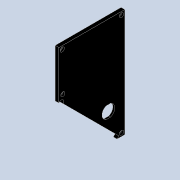
# Autodesk Inventor part: Operator Junction Box Side Panel
Saved by Autodesk Inventor 2022 (Build 260153000, 153)
## iProperties
Created: 2022-01-14
Part Number: Operator Junction Box Side Panel
Material: Generic
Document SubType Name: Modeling
Designer: Coy
Density: 1 g/cm^3
Appearance: Anodized - Black
Author: Coy
Autodesk Inventor part; units mm, degrees
ref_plane "YZ Plane" through (0, 0, 0) normal (1, 0, 0) x (0, 1, 0)
ref_plane "XZ Plane" through (0, 0, 0) normal (0, 1, 0) x (-1, 0, 0)
ref_plane "XY Plane" through (0, 0, 0) normal (0, 0, 1) x (1, 0, 0)
sketch "Sketch1" plane through (0, 0, 0) normal (1, 0, 0) x (0, 1, 0)
  circle A0 centre (7.0357, 7.0379) radius 4.5 construction
  circle A1 centre (222.967, 132.9623) radius 4.5 construction
  arc A2 (216.9926, 130.402) -> (220.4062, 126.988) centre (222.967, 132.9623) ccw construction
  arc A3 (226.4665, 117.7965) -> (220.4062, 126.988) centre (216.4665, 117.7968) ccw construction
  line L0 (226.4665, 117.7965) -> (226.4629, 22.2035) construction
  arc A4 (220.402, 13.0124) -> (226.4629, 22.2035) centre (216.4629, 22.2039) ccw construction
  arc A5 (220.402, 13.0124) -> (216.9879, 9.5985) centre (222.9623, 7.0379) ccw construction
  arc A6 (207.7966, 3.5379) -> (216.9879, 9.5985) centre (207.7966, 13.5379) ccw construction
  line L1 (207.7966, 3.5379) -> (22.2015, 3.5379) construction
  arc A7 (13.0101, 9.5985) -> (22.2015, 3.5379) centre (22.2015, 13.5379) ccw construction
  arc A8 (13.0101, 9.5985) -> (10.3808, 12.6111) centre (7.0357, 7.0379) ccw construction
  line L2 (10.3808, 12.6111) -> (3.8893, 12.6111) construction
  line L3 (3.8893, 12.6111) -> (0, 16.5)
  line L4 (0, 16.5) -> (0, 0)
  line L5 (0, 0) -> (230, 0)
  line L6 (230, 0) -> (230.0052, 140)
  line L7 (230.0052, 140) -> (127.855, 140.0038)
  arc A9 (122.0443, 130.7772) -> (127.855, 140.0038) centre (125.5635, 135.0039) ccw
  line L8 (122.0443, 130.7772) -> (119.5403, 128.2731)
  arc A10 (119.5403, 128.2731) -> (128.6878, 126.5292) centre (125.5635, 135.0039) ccw
  arc A11 (136.9343, 125.9261) -> (128.6878, 126.5292) centre (132.1469, 117.1465) ccw construction
  arc A12 (136.9343, 125.9261) -> (146.2191, 129.5969) centre (140.0462, 131.6328) ccw construction
  arc A13 (155.7163, 136.4648) -> (146.2191, 129.5969) centre (155.716, 126.4648) ccw construction
  line L9 (155.7163, 136.4648) -> (207.8014, 136.4629) construction
  arc A14 (216.9926, 130.402) -> (207.8014, 136.4629) centre (207.801, 126.4629) ccw construction
  circle A15 centre (222.9623, 7.0379) radius 4.5 construction
  circle A16 centre (140.0462, 131.6328) radius 4.5 construction
  arc A17 (184.962, 3.5379) -> (165.0484, 3.5379) centre (175.0052, 35) ccw construction
  line L10 (184.962, 3.5379) -> (226.4622, 3.5379) construction
  line L11 (226.4622, 3.5379) -> (226.4634, 35.0003) construction
  arc A18 (223.4634, 32.0004) -> (226.4634, 35.0003) centre (223.4634, 35.0004) ccw construction
  line L12 (223.4634, 32.0004) -> (213.4634, 32.0004) construction
  arc A19 (213.4634, 38.0004) -> (213.4634, 32.0004) centre (213.4634, 35.0004) ccw construction
  line L13 (213.4634, 38.0004) -> (223.4634, 38.0004) construction
  arc A20 (226.4634, 35.0003) -> (223.4634, 38.0004) centre (223.4634, 35.0004) ccw construction
  line L14 (226.4634, 35.0003) -> (226.4647, 70.0003) construction
  arc A21 (223.4647, 67.0004) -> (226.4647, 70.0003) centre (223.4647, 70.0004) ccw construction
  line L15 (223.4647, 67.0004) -> (213.4647, 67.0004) construction
  arc A22 (213.4647, 73.0004) -> (213.4647, 67.0004) centre (213.4647, 70.0004) ccw construction
  line L16 (213.4647, 73.0004) -> (223.4647, 73.0004) construction
  arc A23 (226.4647, 70.0003) -> (223.4647, 73.0004) centre (223.4647, 70.0004) ccw construction
  line L17 (226.4647, 70.0003) -> (226.466, 105.0003) construction
  arc A24 (223.466, 102.0004) -> (226.466, 105.0003) centre (223.466, 105.0004) ccw construction
  line L18 (223.466, 102.0004) -> (213.466, 102.0004) construction
  arc A25 (213.466, 108.0004) -> (213.466, 102.0004) centre (213.466, 105.0004) ccw construction
  line L19 (213.466, 108.0004) -> (223.466, 108.0004) construction
  arc A26 (226.466, 105.0003) -> (223.466, 108.0004) centre (223.466, 105.0004) ccw construction
  line L20 (226.466, 105.0003) -> (226.4672, 136.4622) construction
  line L21 (226.4672, 136.4622) -> (145.4199, 136.4652) construction
  arc A27 (145.4199, 136.4652) -> (133.0261, 129.9155) centre (145.4194, 121.4652) ccw construction
  arc A28 (119.5403, 128.2731) -> (133.0261, 129.9155) centre (125.5635, 135.0039) ccw construction
  line L22 (119.5403, 128.2731) -> (3.8893, 12.6111)
  line L23 (3.8893, 12.6111) -> (3.5357, 12.9646)
  line L24 (3.5357, 12.9646) -> (3.5357, 3.5379) construction
  line L25 (3.5357, 3.5379) -> (165.0484, 3.5379) construction
  circle A29 centre (7.0357, 7.0379) radius 2.75
  circle A30 centre (222.9623, 7.0379) radius 2.75
  circle A31 centre (222.967, 132.9623) radius 2.75
  circle A32 centre (140.0462, 131.6328) radius 2.75
  dimension "d0" = 5.5
  dimension "d1" = 5.5
  dimension "d2" = 5.5
  dimension "d3" = 5.5
  constraints: 52 end point, 50 point on circle, 33 centre point, 4 coincident
  measures "d0" diameter of A29
  measures "d1" diameter of A30
  measures "d2" diameter of A31
  measures "d3" diameter of A32
extrude "Extrusion1" add sketch "Sketch1" along normal blind 4
sketch "Sketch2" plane through (4, 0, 0) normal (1, 0, 0) x (0, 0, -1)
  line L0 (0, 0) -> (0, 230) projected
  line L1 (0, 230) -> (-140, 230.0052) projected
  line L2 (-140, 230.0052) -> (-140.0038, 127.855) projected
  arc A0 (-130.7772, 122.0443) -> (-140.0038, 127.855) centre (-135.0039, 125.5635) ccw projected
  line L3 (-130.7772, 122.0443) -> (-12.6111, 3.8893) projected
  line L4 (-12.6111, 3.8893) -> (-16.5, 0) projected
  line L5 (-16.5, 0) -> (0, 0) projected
  circle A1 centre (-7.0379, 7.0357) radius 2.75 projected
  circle A2 centre (-7.0379, 222.9623) radius 2.75 projected
  circle A3 centre (-132.9623, 222.967) radius 2.75 projected
  circle A4 centre (-131.6328, 140.0462) radius 2.75 projected
  circle A5 centre (-131.6328, 140.0462) radius 2.75 projected
  circle A6 centre (-131.6328, 140.0462) radius 4.5
  circle A7 centre (-132.9623, 222.967) radius 2.75 projected
  circle A8 centre (-132.9623, 222.967) radius 4.5
  circle A9 centre (-7.0379, 222.9623) radius 4.5
  circle A10 centre (-7.0379, 7.0357) radius 2.75 projected
  circle A11 centre (-7.0379, 7.0357) radius 4.5
  dimension "d6" = 9
  dimension "d7" = 9
  dimension "d8" = 9
  dimension "d9" = 9
  constraints: 4 centre point, 4 coincident
  measures "d6" diameter of A6
  measures "d7" diameter of A8
  measures "d8" diameter of A9
  measures "d9" diameter of A11
extrude "Extrusion2" add sketch "Sketch2" along normal blind 4 contours L5 L4 L3 A0 L2 L1 L0
sketch "Sketch3" plane through (8, 0, 0) normal (1, 0, 0) x (0, 0, -1)
  line L0 (0, 0) -> (0, 230) construction
  line L1 (0, 60) -> (-140.0064, 60.0052) construction
  line L2 (-140, 230.0052) -> (-140.0038, 127.855) construction
  line L3 (-127.855, 140.0038) -> (-230.0052, 140) construction
  line L4 (-210.0052, 140.0007) -> (-210.0052, 0) construction
  line L5 (-230, 0) -> (0, 0) construction
  circle A0 centre (-35, 60.0013) radius 13.5
  line L6 (-57.0351, 47.3513) -> (-57.0351, 72.6513)
  line L7 (-57.0351, 72.6513) -> (-14.4833, 72.6513)
  line L8 (-14.4833, 72.6513) -> (-14.4833, 47.3513)
  line L9 (-14.4833, 47.3513) -> (-57.0351, 47.3513)
  line L10 (-3.55, 0) -> (-3.55, 230) construction
  point P0 (-187.6552, 39.7146)
  point P1 (-187.6552, 30.2854)
  point P2 (-162.3552, 30.2854)
  point P3 (-162.3552, 39.7146)
  point P4 (-39.7146, 47.3513)
  point P5 (-30.2854, 47.3513)
  point P6 (-30.2854, 72.6513)
  point P7 (-39.7146, 72.6513)
  dimension "d12" = 60
  dimension "d13" = 20
  dimension "d14" = 27
  dimension "d17" = 25.3
  dimension "d18" = 0.85
  dimension "d19" = 3.55
  dimension "d20" = 22.0352
  dimension "d21" = 42.5518
  dimension "d22" = 21.5
  constraints: 18 end point, 4 point on line, 3 parallel, 2 perpendicular, 1 centre point, 1 vertical
  measures "d12" distance from line of L0.start L1
  measures "d13" distance from line of L3.end L4
  measures "d14" diameter of A0
  measures "d17" distance of L6.start L6.end
  measures "d18" distance edge to line of A0 L7
  measures "d19" distance between parallel lines of L0 L10
  measures "d20" distance from line of A0.centre L6
  measures "d21" distance of L6.end L7.end
  measures "d22" distance edge to line of A0 L0
extrude "Extrusion3" cut sketch "Sketch3" against normal up to next contours A0 L9 L7
sketch "Sketch4" plane through (0, 0, 0) normal (-1, 0, 0) x (0, 0, 1)
  line L0 (30.2854, 72.6513) -> (39.7146, 72.6513) construction
  line L1 (35, 72.6513) -> (35, 47.3513) construction
  line L2 (30.2854, 47.3513) -> (39.7146, 47.3513) construction
  circle A0 centre (35, 60.0013) radius 18.5
  point P0 (0, 0)
  dimension "d25" = 37
  constraints: 3 midpoint, 2 end point, 1 centre point
  measures "d25" diameter of A0
extrude "Extrusion4" cut sketch "Sketch4" against normal blind 4
fillet "Fillet1" radius 4 1 edges at (0, 60.0013, 16.5)
equation "\"d1\" = d0"
equation "\"d2\" = d0"
equation "\"d3\" = d0"
equation "\"d7\" = d6"
equation "\"d8\" = d6"
equation "\"d9\" = d6"
equation "\"d18\" = -0.5 * d17 + 0.5 * d14"
body "Solid1"
